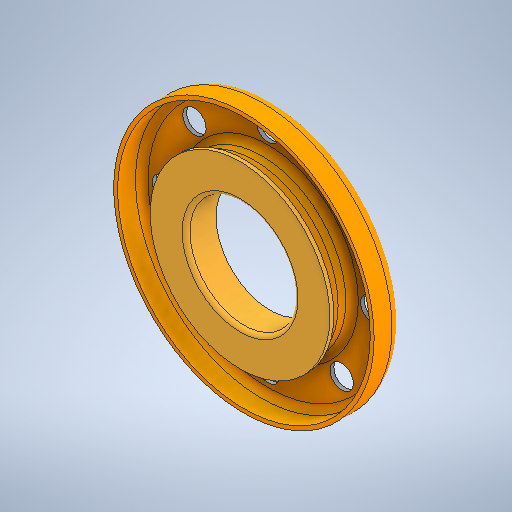
# Autodesk Inventor part: Stamp flange DIN2642-80
Saved by Autodesk Inventor 2025 (Build 290162010, 162A)
## iProperties
Created: 2023-02-20
Part Number: Stamp flange DIN2642-80
Material: Stainless Steel
Document SubType Name: Modeling
Designer: user
Density: 8 g/cm^3
Appearance: Semi-Polished
Author: user
Autodesk Inventor part; units mm, degrees
ref_plane "YZ Plane" through (0, 0, 0) normal (1, 0, 0) x (0, 1, 0)
ref_plane "XZ Plane" through (0, 0, 0) normal (0, 1, 0) x (-1, 0, 0)
ref_plane "XY Plane" through (0, 0, 0) normal (0, 0, 1) x (1, 0, 0)
sketch "Sketch1" plane through (0, 0, 0) normal (0, 1, 0) x (-1, 0, 0)
  line L0 (0, 0) -> (0, -38.85397)
  line L1 (-69, 0) -> (-44.45, 0)
  arc A0 (-41.45, -3) -> (-44.45, 0) centre (-44.45, -3) ccw
  line L2 (-41.45, -3) -> (-41.45, -23)
  line L3 (-41.45, -23) -> (-44.45, -23)
  line L4 (-44.45, -23) -> (-44.45, -3)
  arc A1 (-44.45, -3) -> (-44.45, -3) centre (-44.45, -3) ccw
  line L5 (-44.45, -3) -> (-69, -3)
  line L6 (-69, -3) -> (-69, 0)
  point P0 (-56.725, 0)
  dimension "H_cllr" = 23
  dimension "D_ext_tube" = 88.9
  dimension "D_ext_clllr" = 138
  dimension "d26" = 3
  constraints: 14 end point, 6 perpendicular, 4 tangent, 2 centre point, 2 coincident with centre, 2 point on circle, 1 concentric, 1 horizontal, 1 horizontal alignment, 1 midpoint, 1 vertical
  measures "H_cllr" distance from line of L0.start L3
  measures "D_ext_tube" diameter of L4 L0
  measures "D_ext_clllr" diameter of L6 L0
  measures "d26" distance of L2.end L3.end
sketch "Sketch1 outline for Revolution1" plane through (0, 0, 0) normal (0, 1, 0) x (-1, 0, 0)
  arc A0 (-41.45, -3) -> (-44.45, 0) centre (-44.45, -3) ccw
  line L0 (-41.45, -23) -> (-41.45, -3)
  line L1 (-44.45, -23) -> (-41.45, -23)
  line L2 (-44.45, -3) -> (-44.45, -23)
  line L3 (-69, -3) -> (-44.45, -3)
  line L4 (-69, 0) -> (-69, -3)
  line L5 (-44.45, 0) -> (-69, 0)
revolve "Revolution1" add sketch "Sketch1 outline for Revolution1" angle 360 about axis through (0, 0, 0) along (0, 0, -1)
sketch "Sketch2" plane through (0, 0, 0) normal (0, 1, 0) x (-1, 0, 0)
  line L0 (0, 0) -> (0, -50.951284)
  line L1 (-47, -6) -> (-56.6875, -6)
  arc A0 (-56.6875, -6) -> (-61.5, -10.8125) centre (-56.6875, -10.8125) ccw
  line L2 (-61.5, -10.8125) -> (-61.5, -16.6875)
  arc A1 (-69.3125, -24.5) -> (-61.5, -16.6875) centre (-69.3125, -16.6875) ccw
  line L3 (-69.3125, -24.5) -> (-92.1875, -24.5)
  arc A2 (-100, -16.6875) -> (-92.1875, -24.5) centre (-92.1875, -16.6875) ccw
  line L4 (-100, -16.6875) -> (-100, -3)
  line L5 (-100, -3) -> (-97, -3)
  line L6 (-97, -3) -> (-97, -16.6875)
  arc A3 (-97, -16.6875) -> (-92.1875, -21.5) centre (-92.1875, -16.6875) ccw
  line L7 (-92.1875, -21.5) -> (-69.3125, -21.5)
  arc A4 (-69.3125, -21.5) -> (-64.5, -16.6875) centre (-69.3125, -16.6875) ccw
  line L8 (-64.5, -16.6875) -> (-64.5, -10.8125)
  arc A5 (-56.6875, -3) -> (-64.5, -10.8125) centre (-56.6875, -10.8125) ccw
  line L9 (-56.6875, -3) -> (-47, -3)
  line L10 (-47, -3) -> (-47, -6)
  point P0 (-98.5, -3)
  point P1 (-51.84375, -3)
  dimension "d8" = 3
  dimension "Thknss_lpd" = 3
  dimension "d10" = 4.8125
  dimension "H_lpd" = 21.5
  dimension "D_ext_lpd" = 200
  dimension "d_inn_lpd" = 94
  dimension "d2_inn_lpd" = 123
  dimension "d23" = 38.5
  constraints: 22 end point, 12 point on circle, 12 tangent, 8 perpendicular, 6 centre point, 3 concentric, 2 equal radius, 2 midpoint, 2 point on line, 1 horizontal, 1 horizontal alignment, 1 vertical
  measures "d8" distance from line of L0.start L9
  measures "Thknss_lpd" distance of L9.end L1.start
  measures "d10" radius of A0
  measures "H_lpd" distance between parallel lines of L5 L3
  measures "D_ext_lpd" diameter of L4 L0
  measures "d_inn_lpd" diameter of L10 L0
  measures "d2_inn_lpd" diameter of L2 L0
  measures "d23" distance between parallel lines of L4 L2
revolve "Revolution2" add sketch "Sketch2" angle 360 about axis through (0, 0, 0) along (0, 0, -1)
sketch "Sketch3" plane through (0, 0, 0) normal (0, 0, 1) x (1, 0, 0)
  circle A0 centre (80, 0) radius 9
  line L0 (0, 0) -> (0, 123.830608)
  dimension "hl_d" = 18
  dimension "D_hl_c" = 160
  constraints: 2 end point, 1 centre point, 1 horizontal alignment, 1 vertical
  measures "hl_d" diameter of A0
  measures "D_hl_c" diameter of A0.centre L0
extrude "Extrusion1" cut sketch "Sketch3" against normal through all
pattern_circular "Circular Pattern1" count 8 over 360 about axis through (0, 0, -10) along (0, 0, 1) of "Extrusion1"
equation "\"d26\" = Thknss_lpd"
equation "\"d8\" = Thknss_cllr"
equation "\"d10\" = 0.125 * d23"
equation "\"Thknss_cllr\" = 3"
body "Solid1"
